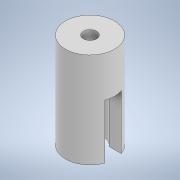
# Autodesk Inventor part: mini fidget foot
Saved by Autodesk Inventor 2022.4 (Build 264492010, 492A)
## iProperties
Created: 2023-03-29
Part Number: mini fidget foot
Material: Generic
Document SubType Name: Modeling
Designer: tmass
Density: 1 g/cm^3
Appearance: Default
Author: tmass
Autodesk Inventor part; units mm, degrees
ref_plane "YZ Plane" through (0, 0, 0) normal (1, 0, 0) x (0, 1, 0)
ref_plane "XZ Plane" through (0, 0, 0) normal (0, 1, 0) x (-1, 0, 0)
ref_plane "XY Plane" through (0, 0, 0) normal (0, 0, 1) x (1, 0, 0)
sketch "Sketch1" plane through (0, 0, 0) normal (0, 0, 1) x (1, 0, 0)
  line L0 (0, 17.5) -> (9, 17.5)
  line L1 (9, 17.5) -> (9, -17.5)
  line L2 (9, -17.5) -> (0, -17.5)
  line L3 (0, -17.5) -> (0, 17.5)
  line L4 (0, 7.5) -> (2.45, 7.5)
  line L5 (2.45, 7.5) -> (2.45, 17.5)
  line L6 (2.45, 17.5) -> (0, 17.5)
  line L7 (0, 17.5) -> (0, 7.5)
  line L8 (0, 7.5) -> (5, 7.5)
  line L9 (5, 7.5) -> (5, -17.5)
  line L10 (5, -17.5) -> (0, -17.5)
  line L11 (0, -17.5) -> (0, 7.5)
  point P0 (0, 0)
  dimension "d0" = 9
  dimension "d1" = 35
  dimension "d2" = 17.5
  dimension "d3" = 10
  dimension "d4" = 2.45
  dimension "d5" = 5
  constraints: 24 end point, 6 parallel, 3 horizontal, 3 perpendicular, 3 point on line, 1 midpoint
  measures "d0" distance of L0.start L0.end
  measures "d1" distance of L0.end L1.end
  measures "d2" distance from line of L0 point (0, 0)
  measures "d3" distance of L4.end L5.end
  measures "d4" distance between parallel lines of L3 L5
  measures "d5" distance of L9.end L10.end
revolve "Revolution1" add sketch "Sketch1" angle 360 about axis through (0, -17.5, 0) along (0, 1, 0) contours L0 L1 L2 L9 L8 L5
sketch "Sketch2" plane through (0, 0, 0) normal (1, 0, 0) x (0, 1, 0)
  line L0 (-17.5, 5) -> (-17.5, -5) projected
  line L1 (2.5, 3) -> (-17.5, 3)
  line L2 (-17.5, 3) -> (-17.5, -3)
  line L3 (-17.5, -3) -> (2.5, -3)
  line L4 (2.5, -3) -> (2.5, 3)
  line L5 (-17.5, 5) -> (7.5, 5) projected
  line L6 (-17.5, -5) -> (7.5, -5) projected
  line L7 (7.5, 5) -> (7.5, -5) projected
  point P0 (2.5, 0)
  dimension "d7" = 2
  dimension "d8" = 2
  dimension "d11" = 5
  constraints: 8 end point, 2 parallel, 1 horizontal, 1 midpoint, 1 perpendicular, 1 point on line
  measures "d7" distance between parallel lines of L5 L1
  measures "d8" distance between parallel lines of L6 L3
  measures "d11" distance between parallel lines of L4 L7
extrude "Extrusion1" cut sketch "Sketch2" along normal through all both and the other way through all contours L1 L4 L3 L0
equation "\"d2\" = 0.5 * d1"
body "Solid1"
